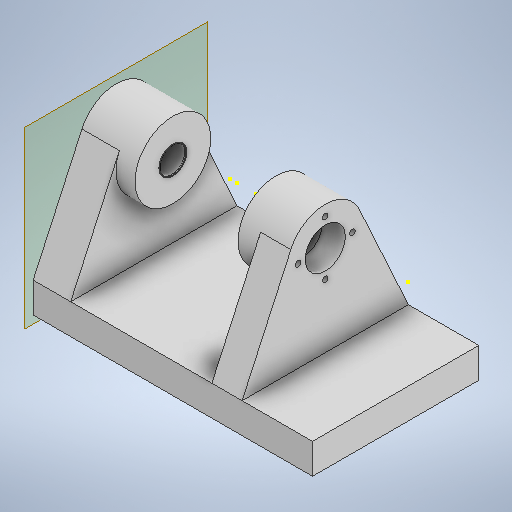
# Autodesk Inventor part: podstawa
Saved by Autodesk Inventor 2025 (Build 290162000, 162)
## iProperties
Created: 2025-05-19
Part Number: podstawa
Material: Ogólny
Document SubType Name: Modeling
Designer: marci
Density: 1 g/cm^3
Appearance: Domyślna
Mass: 615038 g
Surface Area: 81215.4 cm^2
Volume: 615038 cm^3
Author: marci
Autodesk Inventor part; units mm, degrees
ref_plane "YZ Plane" through (0, 0, 0) normal (1, 0, 0) x (0, 1, 0)
ref_plane "XZ Plane" through (0, 0, 0) normal (0, 1, 0) x (-1, 0, 0)
ref_plane "XY Plane" through (0, 0, 0) normal (0, 0, 1) x (1, 0, 0)
sketch "Szkic1" plane through (0, 0, 0) normal (0, 0, 1) x (1, 0, 0)
  line L0 (-172.0995, -130.735) -> (1627.9005, -130.735)
  line L1 (1627.9005, -130.735) -> (1627.9005, -330.735)
  line L2 (1627.9005, -330.735) -> (-172.0995, -330.735)
  line L3 (-172.0995, -330.735) -> (-172.0995, -130.735)
  dimension "d6" = 1800
  dimension "d7" = 200
  constraints: 8 end point, 2 parallel, 1 horizontal, 1 perpendicular
  measures "d6" distance of L1.end L2.end
  measures "d7" distance of L0.end L1.end
extrude "Wyciągnięcie proste1" add sketch "Szkic1" along normal blind 1100
sketch "Szkic2" plane through (-172.0995, -130.735, 0) normal (0, 1, 0) x (1, 0, 0)
  point P0 (172.0995, 0)
sketch "Szkic3" plane through (-172.0995, -130.735, 0) normal (0, 1, 0) x (1, 0, 0)
  line L0 (0, 0) -> (1800, 0) projected
  line L1 (0, -1100) -> (1800, -1100) projected
  line L2 (0, 0) -> (200, 0)
  line L3 (200, 0) -> (200, -1100)
  line L4 (200, -1100) -> (0, -1100)
  line L5 (0, -1100) -> (0, 0)
  line L6 (1800, 0) -> (1700, 0)
  line L7 (1700, -1100) -> (1800, -1100)
  line L8 (1334, 0) -> (1134, 0)
  line L9 (1134, 0) -> (1134, -1100)
  line L10 (1134, -1100) -> (1334, -1100)
  line L11 (1334, -1100) -> (1334, 0)
  line L12 (100, 0) -> (100, -1100)
  line L13 (1234, 0) -> (1234, -1100) construction
  point P0 (172.0995, 0)
  point P1 (1134, 0)
  dimension "d10" = 200
  dimension "d15" = 200
  dimension "d21" = 934
  constraints: 24 end point, 5 parallel, 4 midpoint, 4 point on line, 3 horizontal, 2 perpendicular
  measures "d10" distance of L3.end L4.end
  measures "d15" distance of L10.end L9.end
  measures "d21" distance between parallel lines of L9 L3
extrude "Wyciągnięcie proste2" add sketch "Szkic3" along normal blind 1200 contours L0 L12 L1 L5 | L0 L3 L1 L12 | L0 L11 L1 L9
sketch "Szkic6" plane through (27.9005, -130.735, 1100) normal (1, 0, 0) x (0, 0, -1)
  line L0 (0, 1200) -> (1100, 1200) projected
  line L1 (550, 1200) -> (550, 0)
  line L2 (1100, 0) -> (0, 0) projected
  line L3 (0, 0) -> (0, 1200) projected
  line L4 (0, 600) -> (1100, 600)
  line L5 (1100, 0) -> (1100, 1200) projected
  circle A0 centre (550, 600) radius 85
  point P0 (1100, 130.735)
  dimension "d23" = 170
  constraints: 5 midpoint, 4 end point, 1 centre point
  measures "d23" diameter of A0
extrude "Wyciągnięcie proste4" cut sketch "Szkic6" along normal blind 982 and the other way blind 46 contours A0 L4 L1 | L1 L4 A0 | L4 L1 A0 | L4 A0 L1
sketch "Szkic7" plane through (1161.9005, -130.735, 1100) normal (1, 0, 0) x (0, 0, -1)
  point P0 (1100, 130.735)
sketch "Szkic8" plane through (1161.9005, -130.735, 1100) normal (1, 0, 0) x (0, 0, -1)
  circle A0 centre (550, 600) radius 85 projected
  circle A1 centre (550, 600) radius 132
  point P0 (1100, 130.735)
  dimension "d28" = 264
  constraints: 1 centre point, 1 coincident
  measures "d28" diameter of A1
extrude "Wyciągnięcie proste5" cut sketch "Szkic8" against normal up to surface (152 mm away) contours A0 | A1
sketch "Szkic9" plane through (-172.0995, -330.735, 0) normal (-1, 0, 0) x (0, 0, 1)
  circle A0 centre (550, 800) radius 85 projected
  circle A1 centre (550, 800) radius 132
  point P0 (0, 330.735)
  constraints: 1 centre point, 1 coincident
extrude "Wyciągnięcie proste6" cut sketch "Szkic9" against normal up to surface (154 mm away) contours A0 | A1
sketch "Szkic10" plane through (1161.9005, -130.735, 1100) normal (1, 0, 0) x (0, 0, -1)
  line L0 (1100, 1200) -> (0, 1200) projected
  line L1 (1100, 0) -> (0, 0) projected
  line L2 (0, -200) -> (0, 1200) projected
  circle A0 centre (550, 600) radius 250
  line L3 (0, 0) -> (322.7328, 704.1616)
  line L4 (1100, 0) -> (777.2672, 704.1616)
  line L5 (0, 0) -> (0, 1200)
  line L6 (0, 1200) -> (1100, 1200)
  line L7 (1100, -200) -> (1100, 1200) projected
  line L8 (1100, 1200) -> (1100, 0)
  point P0 (1100, 130.735)
  dimension "d33" = 500
  constraints: 10 end point, 3 collinear, 2 point on circle, 2 tangent, 1 centre point
  measures "d33" diameter of A0
extrude "Wyciągnięcie proste7" cut sketch "Szkic10" against normal through all contours L7 L4 A0 L3 L2 L0
sketch "Szkic11" plane through (-172.0995, -330.735, 0) normal (-1, 0, 0) x (0, 0, 1)
  circle A0 centre (550, 800) radius 132
  circle A1 centre (550, 800) radius 85 projected
  circle A2 centre (550, 800) radius 250
  line L0 (0, 200) -> (1100, 200) projected
  line L1 (0, 0) -> (1100, 0)
  line L2 (1100, 0) -> (1100, 200)
  line L3 (1100, 200) -> (0, 200)
  line L4 (0, 200) -> (0, 0)
  line L5 (1100, 200) -> (777.2672, 904.1616) projected
  line L6 (1100, 200) -> (777.2672, 904.1616)
  line L7 (322.7328, 904.1616) -> (0, 200) projected
  line L8 (0, 200) -> (322.7328, 904.1616)
  point P0 (0, 330.735)
  constraints: 12 end point, 4 equal length, 2 centre point, 2 tangent, 1 coincident, 1 horizontal, 1 perpendicular
extrude "Wyciągnięcie proste8" add sketch "Szkic11" along normal blind 48 contours A2 | A2 L5 L0 L7 | L2 L1 L4 L0
sketch "Szkic12" plane through (-220.0995, -330.735, 0) normal (-1, 0, 0) x (0, 0, 1)
  point P0 (0, 330.735)
sketch "Szkic13" plane through (-18.0995, 469.265, 550) normal (-1, 0, 0) x (0, 0, 1)
  point P0 (-550, -469.265)
ref_plane "Płaszczyzna konstrukcyjna1" through (-220.0995, -330.735, 0) normal (-1, 0, 0) x (0, 0, 1)
sketch "Szkic14" plane through (-220.0995, -330.735, 0) normal (-1, 0, 0) x (0, 0, 1)
  point P0 (0, 330.735)
sketch "Szkic15" plane through (-220.0995, -330.735, 0) normal (-1, 0, 0) x (0, 0, 1)
  point P0 (0, 330.735)
sketch "Szkic16" plane through (-220.0995, -330.735, 0) normal (-1, 0, 0) x (0, 0, 1)
  circle A0 centre (550, 980) radius 18
  point P0 (0, 330.735)
  dimension "d39" = 36
  constraints: 1 centre point
  measures "d39" diameter of A0
extrude "Wyciągnięcie proste9" cut sketch "Szkic16" against normal blind 35
sketch "Szkic18" plane through (-220.0995, -330.735, 0) normal (-1, 0, 0) x (0, 0, 1)
  circle A0 centre (550, 620) radius 18
  circle A1 centre (370, 800) radius 18
  point P0 (0, 330.735)
  dimension "d43" = 36
  dimension "d44" = 36
  constraints: 2 centre point
  measures "d43" diameter of A0
  measures "d44" diameter of A1
extrude "Wyciągnięcie proste10" cut sketch "Szkic18" against normal blind 35
thread "Gwint1" size "M36x4" class "6H" standard "ANSI Metric M Profile" full length
thread "Gwint2" size "M36x4" class "6H" standard "ANSI Metric M Profile" full length
thread "Gwint3" size "M36x4" class "6H" standard "ANSI Metric M Profile" full length
sketch "Szkic19" plane through (-220.0995, -330.735, 0) normal (-1, 0, 0) x (0, 0, 1)
  circle A0 centre (730, 800) radius 18
  point P0 (0, 330.735)
  dimension "d57" = 36
  constraints: 1 centre point
  measures "d57" diameter of A0
extrude "Wyciągnięcie proste12" cut sketch "Szkic19" against normal blind 35
thread "Gwint5" size "M36x4" class "6H" standard "ANSI Metric M Profile" full length
sketch "Szkic20" plane through (27.9005, -130.735, 1100) normal (1, 0, 0) x (0, 0, -1)
  point P0 (1100, 130.735)
sketch "Szkic26" plane through (961.9005, -130.735, 0) normal (-1, 0, 0) x (0, 0, 1)
  circle A0 centre (550, 600) radius 85 projected
  circle A1 centre (550, 600) radius 250
  point P0 (0, 130.735)
  constraints: 1 centre point, 1 coincident
extrude "Wyciągnięcie proste15" add sketch "Szkic26" along normal blind 126
sketch "Szkic27" plane through (835.9005, 469.265, 550) normal (-1, 0, 0) x (0, 0, 1)
  circle A0 centre (0, 0) radius 87
  circle A1 centre (0, 0) radius 92
  point P0 (-550, -469.265)
  dimension "d71" = 174
  dimension "d72" = 184
  constraints: 2 centre point, 1 coincident
  measures "d71" diameter of A0
  measures "d72" diameter of A1
extrude "Wyciągnięcie proste16" cut sketch "Szkic27" against normal blind 8
sketch "Szkic28" plane through (-220.0995, -330.735, 0) normal (-1, 0, 0) x (0, 0, 1)
  point P0 (0, 330.735)
sketch "Szkic29" plane through (1161.9005, -130.735, 1100) normal (1, 0, 0) x (0, 0, -1)
  circle A0 centre (550, 780) radius 18 projected
  circle A1 centre (550, 780) radius 18
  circle A2 centre (730, 600) radius 18 projected
  circle A3 centre (730, 600) radius 18
  circle A4 centre (550, 420) radius 18 projected
  circle A5 centre (550, 420) radius 18
  circle A6 centre (370, 600) radius 18 projected
  circle A7 centre (370, 600) radius 18
  point P0 (1100, 130.735)
  dimension "d75" = 36
  dimension "d76" = 36
  dimension "d77" = 36
  dimension "d78" = 36
  constraints: 4 centre point, 4 coincident
  measures "d75" diameter of A1
  measures "d76" diameter of A3
  measures "d77" diameter of A5
  measures "d78" diameter of A7
extrude "Wyciągnięcie proste17" cut sketch "Szkic29" against normal blind 35
thread "Gwint6" size "M36x4" class "6H" standard "ANSI Metric M Profile" full length
thread "Gwint7" size "M36x4" class "6H" standard "ANSI Metric M Profile" full length
thread "Gwint8" size "M36x4" class "6H" standard "ANSI Metric M Profile" full length
thread "Gwint9" size "M36x4" class "6H" standard "ANSI Metric M Profile" full length
sketch "Szkic30" plane through (27.9005, -130.735, 1100) normal (1, 0, 0) x (0, 0, -1)
  circle A0 centre (550, 600) radius 250
  point P0 (1100, 130.735)
  dimension "d89" = 500
  constraints: 1 centre point
  measures "d89" diameter of A0
extrude "Wyciągnięcie proste18" add sketch "Szkic30" along normal blind 126
sketch "Szkic31" plane through (153.9005, 469.265, 550) normal (1, 0, 0) x (0, 0, -1)
  point P0 (550, -469.265)
sketch "Szkic32" plane through (153.9005, 469.265, 550) normal (1, 0, 0) x (0, 0, -1)
  circle A0 centre (0, 0) radius 85 projected
  circle A1 centre (0, 0) radius 85
  point P0 (550, -469.265)
  dimension "d92" = 170
  constraints: 1 centre point, 1 coincident
  measures "d92" diameter of A1
extrude "Wyciągnięcie proste19" cut sketch "Szkic32" against normal blind 400
sketch "Szkic33" plane through (153.9005, 469.265, 550) normal (1, 0, 0) x (0, 0, -1)
  circle A0 centre (0, 0) radius 87
  circle A1 centre (0, 0) radius 92
  point P0 (550, -469.265)
  dimension "d95" = 174
  dimension "d96" = 184
  constraints: 2 centre point, 1 coincident
  measures "d95" diameter of A0
  measures "d96" diameter of A1
extrude "Wyciągnięcie proste20" cut sketch "Szkic33" against normal blind 8
